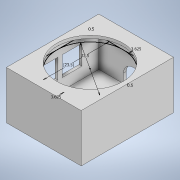
# Autodesk Inventor part: carcasaXeotype_COLOR
Saved by Autodesk Inventor 2020 (Build 240168000, 168)
## iProperties
Created: 2021-04-10
Part Number: carcasaXeotype_COLOR
Material: Generic
Document SubType Name: Modeling
Designer: Vlasciar
Density: 1 g/cm^3
Appearance: Default
Author: Vlasciar
Autodesk Inventor part; units mm, degrees
ref_plane "YZ Plane" through (0, 0, 0) normal (1, 0, 0) x (0, 1, 0)
ref_plane "XZ Plane" through (0, 0, 0) normal (0, 1, 0) x (-1, 0, 0)
ref_plane "XY Plane" through (0, 0, 0) normal (0, 0, 1) x (1, 0, 0)
sketch "Sketch1" plane through (0, 0, 0) normal (0, 1, 0) x (-1, 0, 0)
  line L0 (-13.25, -16.375) -> (13.25, -16.375)
  line L1 (13.25, -16.375) -> (13.25, 16.375)
  line L2 (13.25, 16.375) -> (-13.25, 16.375)
  line L3 (-13.25, 16.375) -> (-13.25, -16.375)
  line L4 (-13.25, -16.375) -> (13.25, 16.375) construction
  line L5 (13.25, -16.375) -> (-13.25, 16.375) construction
  point P0 (0, 0)
  dimension "d0" = 26.5
  dimension "d1" = 32.75
  constraints: 12 end point, 2 midpoint, 2 parallel, 1 horizontal, 1 perpendicular
  measures "d0" distance of L1.end L2.end
  measures "d1" distance of L0.end L1.end
extrude "Extrusion1" add sketch "Sketch1" along normal blind 3.5 and the other way blind 11.5
shell "Shell1" thickness 1 removed faces 1 at (4.4167, -11.5, 5.4583)
sketch "Sketch2" plane through (0, 3.5, 0) normal (0, 1, 0) x (1, 0, 0)
  line L0 (13.25, 16.375) -> (-13.25, 16.375) projected
  line L1 (-13.25, 16.375) -> (-13.25, -16.375) projected
  line L2 (-13.25, -16.375) -> (13.25, -16.375) projected
  line L3 (13.25, -16.375) -> (13.25, 16.375) projected
  point P0 (0, 0)
extrude "Extrusion2" add sketch "Sketch2" along normal blind 1
sketch "Sketch3" plane through (-12.25, 2.5, -15.375) normal (0, -1, 0) x (1, 0, 0)
  line L0 (24.5, 0) -> (0, 0) projected
  line L1 (24.5, 30.75) -> (24.5, 0) projected
  line L2 (0, 30.75) -> (24.5, 30.75) projected
  line L3 (0, 0) -> (0, 30.75) projected
  line L4 (0.5, 3.625) -> (24, 3.625)
  line L5 (24, 3.625) -> (24, 27.125)
  line L6 (24, 27.125) -> (0.5, 27.125)
  line L7 (0.5, 27.125) -> (0.5, 3.625)
  circle A0 centre (12.25, 15.375) radius 11.75
  dimension "d9" = 0.5
  dimension "d10" = 0.5
  dimension "d11" = 3.625
  dimension "d12" = 3.625
  dimension "d13" = 23.5
  dimension "d14" = 23.5
  constraints: 8 end point, 2 parallel, 1 centre point, 1 coincident, 1 horizontal, 1 perpendicular
  measures "d9" distance between parallel lines of L3 L7
  measures "d10" distance between parallel lines of L1 L5
  measures "d11" distance between parallel lines of L2 L6
  measures "d12" distance between parallel lines of L0 L4
  measures "d13" distance between parallel lines of L6 L4
  measures "d14" diameter of A0
extrude "Extrusion3" cut sketch "Sketch3" against normal blind 1 contours L7 A0 L4 | A0 L5 L4 | A0 | L7 L6 A0 | A0 L6 L5
extrude "Extrusion4" cut sketch "Sketch3" against normal blind 2 contours A0
sketch "Sketch4" plane through (-12.25, -11.5, -15.375) normal (0, 0, 1) x (1, 0, 0)
  line L0 (24.5, 0) -> (0, 0) projected
  line L1 (8.75, 6.5) -> (15.75, 6.5)
  line L2 (15.75, 6.5) -> (15.75, 0)
  line L3 (15.75, 0) -> (8.75, 0)
  line L4 (8.75, 0) -> (8.75, 6.5)
  line L5 (8.75, 6.5) -> (15.75, 0) construction
  line L6 (15.75, 6.5) -> (8.75, 0) construction
  circle A0 centre (12.25, 3.25) radius 3.5
  line L7 (15.75, 3.25) -> (15.75, 3.25)
  line L8 (8.75, 3.25) -> (8.75, 3.25)
  point P0 (12.25, 11.5)
  point P1 (12.25, 3.25)
  point P2 (12.25, 0)
  point P3 (12.25, 0)
  point P4 (10.951, 0)
  point P5 (13.549, 0)
  point P6 (15.75, 0)
  point P7 (15.75, 3.25)
  point P8 (8.75, 3.25)
  point P9 (8.75, 0)
  dimension "d19" = 7
  dimension "d20" = 6.5
  dimension "d21" = 7
  dimension "d22" = 3.25
  dimension "d23" = 3.25
  constraints: 16 end point, 7 midpoint, 2 coincident, 2 line through centre, 2 parallel, 2 point on circle, 1 centre point, 1 horizontal, 1 perpendicular, 1 vertical alignment
  measures "d19" distance between parallel lines of L2 L4
  measures "d20" distance of L3.end L1.start
  measures "d21" diameter of A0
  measures "d22" distance between parallel lines of L1 L8
  measures "d23" distance between parallel lines of L1 L7
extrude "Extrusion5" cut sketch "Sketch4" against normal blind 2 contours L0 A0 L2 | A0 L0 | L0 A0 L1 | L0 L4 A0 | L1 A0
sketch "Sketch5" plane through (-13.25, -11.5, -16.375) normal (-1, 0, 0) x (0, 0, 1)
  line L0 (0, 16) -> (32.75, 16) projected
  line L1 (30, 11) -> (3.2984, 11)
  line L2 (7, 11) -> (7, 3)
  line L3 (1, 0) -> (1, 14) projected
  line L4 (7, 4) -> (14, 4)
  line L5 (14, 4) -> (14, 11)
  line L6 (15.5, 11) -> (22.5, 11)
  line L7 (22.5, 11) -> (22.5, 4)
  line L8 (22.5, 4) -> (15.5, 4)
  line L9 (15.5, 4) -> (15.5, 11)
  point P0 (16.375, 11.5)
  dimension "d26" = 5
  dimension "d27" = 6
  dimension "d28" = 7
  dimension "d29" = 7
  dimension "d30" = 7
  dimension "d31" = 7
  dimension "d32" = 1.5
  constraints: 16 end point, 4 point on line, 3 horizontal, 2 parallel, 2 perpendicular, 1 vertical
  measures "d26" distance between parallel lines of L1 L0
  measures "d27" distance between parallel lines of L3 L2
  measures "d28" distance between parallel lines of L4 L1
  measures "d29" distance between parallel lines of L2 L5
  measures "d30" distance between parallel lines of L9 L7
  measures "d31" distance between parallel lines of L8 L1
  measures "d32" distance between parallel lines of L5 L9
extrude "Extrusion6" cut sketch "Sketch5" against normal blind 2
sketch "Sketch6" plane through (0, -11.5, 0) normal (0, -1, 0) x (1, 0, 0)
  line L0 (3.5, -16.375) -> (13.25, -16.375) projected
  line L1 (13.25, -16.375) -> (13.25, 16.375) projected
  line L2 (13.25, 16.375) -> (-13.25, 16.375) projected
  line L3 (-13.25, 16.375) -> (-13.25, -16.375) projected
  line L4 (-13.25, -16.375) -> (-3.5, -16.375) projected
  line L5 (13.25, 16.375) -> (-13.25, 16.375)
  line L6 (-13.25, 16.375) -> (-13.25, -16.375)
  line L7 (-13.25, -16.375) -> (13.25, -16.375)
  line L8 (13.25, -16.375) -> (13.25, 16.375)
  point P0 (0, 0)
  constraints: 8 end point, 2 parallel, 1 horizontal, 1 perpendicular
extrude "Extrusion7" add sketch "Sketch6" along normal blind 1
body "Solid1"
